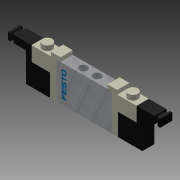
# Autodesk Inventor part: Festo Valve 1764
Saved by Autodesk Inventor 2011 (Build 150239000, 239)
## iProperties
Created: 2010-02-17
Part Number: Festo Valve 1764
Document SubType Name: Modeling
Designer: jgehrig
Density: 1 g/cm^3
Author: jgehrig
Autodesk Inventor part; units mm, degrees
ref_plane "YZ Plane" through (0, 0, 0) normal (1, 0, 0) x (0, 1, 0)
ref_plane "XZ Plane" through (0, 0, 0) normal (0, 1, 0) x (-1, 0, 0)
sketch "Sketch1" plane through (0, 0, 0) normal (0, 0, 1) x (1, 0, 0)
  line L0 (52.6803, 14.9225) -> (52.6803, -13.6525)
  line L1 (52.6803, -13.6525) -> (-38.7597, -13.6525)
  line L2 (-38.7597, -13.6525) -> (-38.7597, 14.9225)
  line L3 (-19.0747, 18.0975) -> (-11.4547, 18.0975)
  line L4 (-11.4547, 18.0975) -> (-11.4547, 14.9225)
  line L5 (-19.0747, 14.9225) -> (-19.0747, 18.0975)
  line L6 (25.3753, 18.0975) -> (32.9953, 18.0975)
  line L7 (32.9953, 18.0975) -> (32.9953, 14.9225)
  line L8 (25.3753, 14.9225) -> (25.3753, 18.0975)
  line L9 (32.9953, 14.9225) -> (52.6803, 14.9225)
  line L10 (-38.7597, 14.9225) -> (-19.0747, 14.9225)
  line L11 (-11.4547, 14.9225) -> (25.3753, 14.9225)
  point P0 (0, 0)
  dimension "d0" = 28.575
  dimension "d1" = 91.44
  dimension "d2" = 7.62
  dimension "d3" = 7.62
  dimension "d4" = 3.175
  dimension "d5" = 3.175
  dimension "d6" = 3.175
  dimension "d7" = 3.175
  dimension "d8" = 19.685
  dimension "d9" = 19.685
  dimension "d10" = 36.83
  constraints: 24 end point, 6 parallel, 5 horizontal, 5 perpendicular
  measures "d0" distance of L1.end L2.end
  measures "d1" distance of L0.end L1.end
  measures "d2" distance of L3.start L3.end
  measures "d3" distance of L6.start L6.end
  measures "d4" distance of L5.start L3.start
  measures "d5" distance of L8.start L6.start
  measures "d6" distance of L6.end L7.end
  measures "d7" distance of L3.end L4.end
  measures "d8" distance between parallel lines of L0 L7
  measures "d9" distance of L2.end L5.start
  measures "d10" distance of L4.end L8.start
extrude "Extrusion1" add sketch "Sketch1" along normal blind 9.525
sketch "Sketch2" plane through (0, 0, 9.525) normal (0, 0, 1) x (1, 0, 0)
  line L0 (-38.7597, 14.9225) -> (-19.0747, 14.9225) projected
  line L1 (52.6803, -13.6525) -> (-38.7597, -13.6525) projected
  line L2 (32.9953, 14.9225) -> (52.6803, 14.9225) projected
  line L3 (32.9953, 18.0975) -> (32.9953, 14.9225) projected
  line L4 (25.3753, 18.0975) -> (32.9953, 18.0975) projected
  line L5 (25.3753, 14.9225) -> (25.3753, 18.0975) projected
  line L6 (-11.4547, 18.0975) -> (-11.4547, 14.9225) projected
  line L7 (-19.0747, 18.0975) -> (-11.4547, 18.0975) projected
  line L8 (-19.0747, 14.9225) -> (-19.0747, 18.0975) projected
  line L9 (-11.4547, 14.9225) -> (-14.6297, 14.9225)
  line L10 (-14.6297, 14.9225) -> (-14.6297, -13.6525)
  line L11 (25.3753, 14.9225) -> (28.5503, 14.9225)
  line L12 (28.5503, 14.9225) -> (28.5503, -13.6525)
  line L13 (33.6303, -13.6525) -> (33.6303, 3.4925)
  line L14 (33.6303, 3.4925) -> (48.2353, 3.4925)
  line L15 (48.2353, 3.4925) -> (48.2353, 14.9225)
  line L16 (-19.7097, -13.6525) -> (-19.7097, 3.4925)
  line L17 (-19.7097, 3.4925) -> (-34.3147, 3.4925)
  line L18 (-34.3147, 3.4925) -> (-34.3147, 14.9225)
  point P0 (0, 0)
  dimension "d13" = 3.175
  dimension "d14" = 3.175
  dimension "d15" = 5.08
  dimension "d16" = 5.08
  dimension "d17" = 19.685
  dimension "d18" = 19.685
  dimension "d19" = 11.43
  dimension "d20" = 11.43
  constraints: 20 end point, 8 perpendicular, 6 point on line, 2 parallel
  measures "d13" distance of L6.end L9.end
  measures "d14" distance of L5.start L11.end
  measures "d15" distance between parallel lines of L13 L12
  measures "d16" distance between parallel lines of L16 L10
  measures "d17" distance between parallel lines of L10 L18
  measures "d18" distance between parallel lines of L15 L12
  measures "d19" distance of L17.end L18.end
  measures "d20" distance of L14.end L15.end
extrude "Extrusion2" add sketch "Sketch2" along normal blind 0.0254
sketch "Sketch3" plane through (0, 0, 0) normal (0, 0, -1) x (-1, 0, 0)
  line L0 (19.0747, 14.9225) -> (38.7597, 14.9225) projected
  line L1 (19.0747, 18.0975) -> (19.0747, 14.9225) projected
  line L2 (11.4547, 18.0975) -> (19.0747, 18.0975) projected
  line L3 (11.4547, 14.9225) -> (11.4547, 18.0975) projected
  line L4 (-25.3753, 18.0975) -> (-25.3753, 14.9225) projected
  line L5 (-32.9953, 18.0975) -> (-25.3753, 18.0975) projected
  line L6 (-32.9953, 14.9225) -> (-32.9953, 18.0975) projected
  line L7 (-52.6803, 14.9225) -> (-32.9953, 14.9225) projected
  line L8 (38.7597, -13.6525) -> (-52.6803, -13.6525) projected
  line L9 (-28.5503, -13.6525) -> (-28.5503, 14.9225) projected
  line L10 (-28.5503, 14.9225) -> (-25.3753, 14.9225) projected
  line L11 (-48.2353, 14.9225) -> (-48.2353, 3.4925) projected
  line L12 (-48.2353, 3.4925) -> (-33.6303, 3.4925) projected
  line L13 (-33.6303, 3.4925) -> (-33.6303, -13.6525) projected
  line L14 (14.6297, 14.9225) -> (14.6297, -13.6525) projected
  line L15 (11.4547, 14.9225) -> (14.6297, 14.9225) projected
  line L16 (34.3147, 3.4925) -> (34.3147, 14.9225) projected
  line L17 (19.7097, 3.4925) -> (34.3147, 3.4925) projected
  line L18 (19.7097, -13.6525) -> (19.7097, 3.4925) projected
  point P0 (0, 0)
extrude "Extrusion3" add sketch "Sketch3" along normal blind 0.0254
sketch "Sketch4" plane through (-38.7597, -13.6525, 0) normal (0, -1, 0) x (1, 0, 0)
  line L0 (72.39, 9.5504) -> (67.31, 9.5504) projected
  line L1 (67.31, 9.525) -> (67.31, 9.5504) projected
  line L2 (67.31, -0.0254) -> (72.39, -0.0254) projected
  line L3 (72.39, 0) -> (72.39, -0.0254) projected
  line L4 (19.685, -0.0254) -> (4.445, -0.0254) projected
  line L5 (27.305, -0.0254) -> (19.685, -0.0254) projected
  line L6 (24.13, -0.0254) -> (27.305, -0.0254) projected
  line L7 (19.05, -0.0254) -> (24.13, -0.0254) projected
  line L8 (4.445, -0.0254) -> (19.05, -0.0254) projected
  line L9 (72.39, 0) -> (72.39, 9.5504)
  line L10 (24.13, -0.0254) -> (24.13, 9.5504)
  line L11 (19.05, -0.0254) -> (19.05, 9.525)
  line L12 (67.31, -0.0254) -> (67.31, 9.525)
  line L13 (91.44, 0) -> (91.44, 9.525) projected
  line L14 (24.13, 0) -> (19.05, 0)
  line L15 (19.05, 9.5504) -> (24.13, 9.525)
  line L16 (24.13, 0) -> (19.05, 0)
  line L17 (19.05, 0) -> (19.05, 9.5504)
  line L18 (19.05, 9.5504) -> (24.13, 9.5504)
  line L19 (24.13, 9.5504) -> (24.13, 0)
  point P0 (38.7597, 0)
  constraints: 20 end point, 4 parallel, 3 perpendicular, 1 horizontal
extrude "Extrusion4" add sketch "Sketch4" along normal blind 0.0254 contours L9 L3 L2 L12 L1 L0 | L11 L17 L15 L10 L14 | L15 L18 L10
sketch "Sketch5" plane through (52.6803, 14.9225, 9.525) normal (0, 1, 0) x (1, 0, 0)
  line L0 (-4.445, 9.5504) -> (-19.685, 9.5504) projected
  line L1 (-19.685, -0.0254) -> (-4.445, -0.0254) projected
  line L2 (-64.135, 0) -> (-27.305, 0) projected
  line L3 (-27.305, 9.525) -> (-27.305, 0) projected
  line L4 (-27.305, 9.525) -> (-64.135, 9.525) projected
  line L5 (-64.135, 9.525) -> (-64.135, 0) projected
  line L6 (-91.44, 0) -> (-86.995, 0) projected
  line L7 (-86.995, 0) -> (-86.995, -0.0254) projected
  line L8 (-86.995, -0.0254) -> (-71.755, -0.0254) projected
  line L9 (-71.755, 9.5504) -> (-71.755, -0.0254) projected
  line L10 (-71.755, 9.5504) -> (-86.995, 9.5504) projected
  line L11 (-86.995, 9.525) -> (-86.995, 9.5504) projected
  line L12 (-86.995, 9.525) -> (-91.44, 9.525) projected
  line L13 (-91.44, 9.525) -> (-91.44, 0) projected
  line L14 (-71.755, 9.5504) -> (-71.755, -0.0254) projected
  line L15 (-27.305, 9.5504) -> (-27.305, -0.0254) projected
  line L16 (-19.685, 9.5504) -> (-19.685, -0.0254) projected
  line L17 (-64.135, 9.5504) -> (-64.135, -0.0254) projected
  line L18 (-4.445, 9.5504) -> (-4.445, -0.0254)
  line L19 (-86.995, -0.0254) -> (-86.995, 9.525)
  point P0 (-52.6803, 9.525)
  constraints: 4 end point, 2 parallel
extrude "Extrusion5" add sketch "Sketch5" along normal blind 0.0254 contours L18 L1 L16 L0 | L19 L11 L10 L9 L8 L7
sketch "Sketch6" plane through (0, 0, 0) normal (0, 0, -1) x (-1, 0, 0)
  line L0 (-52.6803, -13.6525) -> (-52.6803, 14.9225) projected
  line L1 (19.7097, 3.4925) -> (19.7097, -13.6525) projected
  line L2 (38.7597, -13.6525) -> (19.7097, -13.6525) projected
  line L3 (38.7597, 14.9225) -> (38.7597, -13.6525) projected
  line L4 (34.3147, 14.9225) -> (38.7597, 14.9225) projected
  line L5 (34.3147, 14.9225) -> (34.3147, 3.4925) projected
  line L6 (34.3147, 3.4925) -> (19.7097, 3.4925) projected
  line L7 (-62.2053, 14.9225) -> (-52.6803, 14.9225)
  line L8 (-52.6803, 14.9225) -> (-52.6803, 9.2075)
  line L9 (-52.6803, 9.2075) -> (-62.2053, 9.2075)
  line L10 (-62.2053, 9.2075) -> (-62.2053, 14.9225)
  line L11 (38.7597, 14.9225) -> (48.2847, 14.9225)
  line L12 (48.2847, 14.9225) -> (48.2847, 9.2075)
  line L13 (48.2847, 9.2075) -> (38.7597, 9.2075)
  line L14 (38.7597, 9.2075) -> (38.7597, 14.9225)
  point P0 (0, 0)
  dimension "d29" = 9.525
  dimension "d30" = 9.525
  dimension "d31" = 5.715
  dimension "d32" = 5.715
  constraints: 16 end point, 4 parallel, 2 horizontal, 2 perpendicular, 1 point on line
  measures "d29" distance of L7.start L7.end
  measures "d30" distance of L3.start L11.end
  measures "d31" distance of L11.end L12.end
  measures "d32" distance of L9.end L7.start
extrude "Extrusion6" add sketch "Sketch6" against normal blind 9.525 contours L9 L10 L7 L0 | L3 L11 L12 L13
ref_plane "Work Plane1" through (0, 0, 4.7625) normal (0, 0, 1) x (1, 0, 0)
sketch "Sketch7" plane through (0, 0, 4.7625) normal (0, 0, 1) x (1, 0, 0)
  line L0 (-19.7097, 3.4925) -> (-19.7097, -13.6525) projected
  line L1 (-38.7597, -13.6525) -> (-19.7097, -13.6525) projected
  line L2 (-38.7597, 9.2075) -> (-38.7597, -13.6525) projected
  line L3 (-38.7597, 9.2075) -> (-48.2847, 9.2075) projected
  line L4 (-48.2847, 9.2075) -> (-48.2847, 14.9225) projected
  line L5 (-34.3147, 14.9225) -> (-48.2847, 14.9225) projected
  line L6 (-34.3147, 14.9225) -> (-34.3147, 3.4925) projected
  line L7 (-34.3147, 3.4925) -> (-19.7097, 3.4925) projected
  line L8 (48.2353, 3.4925) -> (48.2353, 14.9225) projected
  line L9 (48.2353, 14.9225) -> (62.2053, 14.9225) projected
  line L10 (62.2053, 14.9225) -> (62.2053, 9.2075) projected
  line L11 (62.2053, 9.2075) -> (52.6803, 9.2075) projected
  line L12 (52.6803, -13.6525) -> (52.6803, 9.2075) projected
  line L13 (33.6303, -13.6525) -> (52.6803, -13.6525) projected
  line L14 (33.6303, -13.6525) -> (33.6303, 3.4925) projected
  line L15 (33.6303, 3.4925) -> (48.2353, 3.4925) projected
  line L16 (-48.2847, 13.97) -> (-50.8247, 13.97)
  line L17 (-50.8247, 13.97) -> (-50.8247, 10.16)
  line L18 (-50.8247, 10.16) -> (-48.2847, 10.16)
  line L19 (-48.2847, 10.16) -> (-48.2847, 13.97)
  line L20 (62.2053, 13.97) -> (64.7453, 13.97)
  line L21 (64.7453, 13.97) -> (64.7453, 10.16)
  line L22 (64.7453, 10.16) -> (62.2053, 10.16)
  line L23 (62.2053, 10.16) -> (62.2053, 13.97)
  point P0 (0, 0)
  dimension "d36" = 2.54
  dimension "d37" = 2.54
  dimension "d38" = 3.81
  dimension "d39" = 3.81
  dimension "d40" = 0.9525
  dimension "d41" = 0.9525
  dimension "d42" = 0.9525
  constraints: 16 end point, 4 parallel, 2 horizontal, 2 perpendicular, 2 point on line
  measures "d36" distance of L20.start L20.end
  measures "d37" distance of L16.start L16.end
  measures "d38" distance of L16.end L17.end
  measures "d39" distance of L20.end L21.end
  measures "d40" distance between parallel lines of L9 L20
  measures "d41" distance between parallel lines of L22 L11
  measures "d42" distance between parallel lines of L5 L16
extrude "Extrusion7" add sketch "Sketch7" along normal mid plane 6.35 contours L4 L18 L17 L16 | L20 L21 L22 L10
sketch "Sketch8" plane through (0, 0, 4.7625) normal (0, 0, 1) x (1, 0, 0)
  line L0 (-48.2847, 13.97) -> (-48.2847, 10.16) projected
  line L1 (-50.8247, 13.97) -> (-48.2847, 13.97) projected
  line L2 (-50.8247, 10.16) -> (-50.8247, 13.97) projected
  line L3 (-48.2847, 10.16) -> (-50.8247, 10.16) projected
  line L4 (62.2053, 13.97) -> (64.7453, 13.97) projected
  line L5 (62.2053, 10.16) -> (62.2053, 13.97) projected
  line L6 (64.7453, 10.16) -> (62.2053, 10.16) projected
  line L7 (64.7453, 13.97) -> (64.7453, 10.16) projected
  line L8 (-52.7297, 14.9225) -> (-50.8247, 14.9225)
  line L9 (-50.8247, 14.9225) -> (-50.8247, 9.2075)
  line L10 (-50.8247, 9.2075) -> (-52.7297, 9.2075)
  line L11 (-52.7297, 9.2075) -> (-52.7297, 14.9225)
  line L12 (64.7453, 14.9225) -> (66.6503, 14.9225)
  line L13 (66.6503, 14.9225) -> (66.6503, 9.2075)
  line L14 (66.6503, 9.2075) -> (64.7453, 9.2075)
  line L15 (64.7453, 9.2075) -> (64.7453, 14.9225)
  line L16 (48.2353, 14.9225) -> (62.2053, 14.9225) projected
  line L17 (62.2053, 9.2075) -> (52.6803, 9.2075) projected
  line L18 (-38.7597, 9.2075) -> (-48.2847, 9.2075) projected
  line L19 (-48.2847, 14.9225) -> (-34.3147, 14.9225) projected
  point P0 (0, 0)
  dimension "d45" = 0
  dimension "d46" = 0
  dimension "d47" = 0
  dimension "d48" = 0
  dimension "d49" = 1.905
  dimension "d50" = 5.715
  dimension "d51" = 0
  dimension "d52" = 1.905
  dimension "d53" = 0
  constraints: 16 end point, 4 parallel, 2 horizontal, 2 perpendicular
  measures "d45" distance between parallel lines of L16 L12
  measures "d46" distance between parallel lines of L17 L14
  measures "d47" distance between parallel lines of L18 L10
  measures "d48" distance between parallel lines of L19 L8
  measures "d49" distance of L8.start L8.end
  measures "d50" distance of L10.end L8.start
  measures "d51" distance between parallel lines of L9 L2
  measures "d52" distance of L12.start L12.end
  measures "d53" distance between parallel lines of L7 L15
extrude "Extrusion8" add sketch "Sketch8" along normal mid plane 9.525 contours L2 L9 L10 L11 L8 | L15 L12 L13 L14 L7
sketch "Sketch9" plane through (52.6803, 14.9479, 9.525) normal (0, 1, 0) x (1, 0, 0)
  line L0 (-4.445, 9.5504) -> (-4.445, -0.0254) projected
  line L1 (-19.685, 9.5504) -> (-4.445, 9.5504) projected
  line L2 (-19.685, -0.0254) -> (-19.685, 9.5504) projected
  line L3 (-4.445, -0.0254) -> (-19.685, -0.0254) projected
  circle A0 centre (-12.065, 4.7625) radius 3.81
  circle A1 centre (-79.375, 4.7625) radius 3.81
  point P0 (-52.6803, 9.525)
  dimension "d56" = 7.62
  dimension "d57" = 7.62
  constraints: 2 centre point
  measures "d56" diameter of A0
  measures "d57" diameter of A1
extrude "Extrusion9" add sketch "Sketch9" along normal blind 3.81 contours A0 | A1
sketch "Sketch10" plane through (-14.6297, -13.6525, 9.525) normal (0, -1, 0) x (1, 0, 0)
  line L0 (43.18, -9.525) -> (43.18, 0) projected
  line L1 (0, 0) -> (0, -9.525) projected
  circle A0 centre (10.795, -4.7625) radius 3.175
  circle A1 centre (21.59, -4.7625) radius 3.175
  circle A2 centre (32.385, -4.7625) radius 3.175
  point P0 (14.6297, -9.525)
  dimension "d60" = 6.35
  dimension "d61" = 10.795
  dimension "d62" = 10.795
  dimension "d63" = 10.795
  dimension "d64" = 10.795
  constraints: 3 centre point, 2 equal radius
  measures "d60" diameter of A0
  measures "d61" distance from line of L1 A0.centre
  measures "d62" distance of A1.centre A0.centre
  measures "d63" distance of A1.centre A2.centre
  measures "d64" distance from line of L0 A2.centre
extrude "Extrusion10" cut sketch "Sketch10" against normal blind 10.16
sketch "Sketch11" plane through (-11.4547, 14.9225, 9.525) normal (0, 1, 0) x (1, 0, 0)
  line L0 (36.83, 9.525) -> (36.83, 0) projected
  line L1 (0, 9.525) -> (0, 0) projected
  circle A0 centre (23.8125, 4.7625) radius 3.175
  circle A1 centre (13.0175, 4.7625) radius 3.175
  line L2 (23.8125, 4.7625) -> (36.83, 4.7625)
  line L3 (13.0175, 4.7625) -> (0, 4.7625)
  point P0 (11.4547, 9.525)
  dimension "d67" = 6.35
  dimension "d68" = 10.795
  constraints: 4 end point, 2 centre point, 2 midpoint, 1 collinear, 1 equal radius
  measures "d67" diameter of A0
  measures "d68" distance of L3.start L2.start
extrude "Extrusion11" cut sketch "Sketch11" against normal blind 10.16
sketch "Sketch12" plane through (0, 0, 9.525) normal (0, 0, 1) x (1, 0, 0)
  line L0 (-11.4547, 14.9225) -> (25.3753, 14.9225) projected
  line L1 (-14.6297, 14.9225) -> (-14.6297, -13.6525) projected
  line L2 (28.5503, -13.6525) -> (-14.6297, -13.6525) projected
  line L3 (-10.8197, -9.525) -> (-10.8197, 10.795) construction
  line L4 (-10.8197, 10.795) -> (-6.9164, 10.795) construction
  line L5 (-6.9164, 10.795) -> (-6.9164, -9.525) construction
  line L6 (-6.9164, -9.525) -> (-10.8197, -9.525) construction
  point P0 (0, 0)
  dimension "d72" = 20.32
  dimension "d84" = 3.81
  dimension "d85" = 4.1275
  dimension "d86" = 4.1275
  constraints: 2 other
  measures "d72" distance of L3.start L3.end
  measures "d84" distance between parallel lines of L1 L3
  measures "d85" distance between parallel lines of L0 L4
  measures "d86" distance between parallel lines of L2 L6
decal "Decal1"
body "Solid1"
